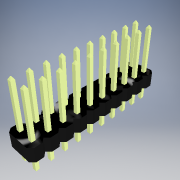
# Autodesk Inventor part: PinHeader-2x10-Male-NoCover
Saved by Autodesk Inventor 2018 (Build 220112000, 112)
## iProperties
Created: 2020-04-19
Part Number: PinHeader-2x10-Male-NoCover
Material: Všeobecné
Document SubType Name: Modeling
Designer: Jozko Mrkvicka
Density: 1 g/cm^3
Appearance: Výchozí
Author: Jozko Mrkvicka
Autodesk Inventor part; units mm, degrees
ref_plane "YZ Plane" through (0, 0, 0) normal (1, 0, 0) x (0, 1, 0)
ref_plane "XZ Plane" through (0, 0, 0) normal (0, 1, 0) x (-1, 0, 0)
ref_plane "XY Plane" through (0, 0, 0) normal (0, 0, 1) x (1, 0, 0)
sketch "Náčrt4" plane through (0, 0, 0) normal (0, 1, 0) x (-1, 0, 0)
  line L0 (4.445, 0) -> (0.635, 0)
  line L1 (0.635, -25.4) -> (4.445, -25.4)
  line L2 (4.445, 0) -> (5.08, -0.635)
  line L3 (5.08, -1.905) -> (4.445, -2.54)
  line L4 (4.445, -2.54) -> (5.08, -3.175)
  line L5 (5.08, -4.445) -> (4.445, -5.08)
  line L6 (4.445, -5.08) -> (5.08, -5.715)
  line L7 (5.08, -6.985) -> (4.445, -7.62)
  line L8 (4.445, -7.62) -> (5.08, -8.255)
  line L9 (5.08, -8.255) -> (5.08, -9.525)
  line L10 (5.08, -9.525) -> (4.445, -10.16)
  line L11 (4.445, -10.16) -> (5.08, -10.795)
  line L12 (5.08, -12.065) -> (4.445, -12.7)
  line L13 (4.445, -12.7) -> (5.08, -13.335)
  line L14 (5.08, -14.605) -> (4.445, -15.24)
  line L15 (4.445, -15.24) -> (5.08, -15.875)
  line L16 (5.08, -17.145) -> (4.445, -17.78)
  line L17 (4.445, -17.78) -> (5.08, -18.415)
  line L18 (5.08, -19.685) -> (4.445, -20.32)
  line L19 (4.445, -20.32) -> (5.08, -20.955)
  line L20 (5.08, -22.225) -> (4.445, -22.86)
  line L21 (4.445, -22.86) -> (5.08, -23.495)
  line L22 (5.08, -24.765) -> (4.445, -25.4)
  line L23 (5.08, -24.765) -> (5.08, -23.495)
  line L24 (5.08, -22.225) -> (5.08, -20.955)
  line L25 (5.08, -19.685) -> (5.08, -18.415)
  line L26 (5.08, -17.145) -> (5.08, -15.875)
  line L27 (5.08, -14.605) -> (5.08, -13.335)
  line L28 (5.08, -12.065) -> (5.08, -10.795)
  line L29 (5.08, -9.525) -> (5.08, -8.255)
  line L30 (5.08, -6.985) -> (5.08, -5.715)
  line L31 (5.08, -4.445) -> (5.08, -3.175)
  line L32 (5.08, -1.905) -> (5.08, -0.635)
  line L33 (0.635, 0) -> (0, -0.635)
  line L34 (0, -1.905) -> (0.635, -2.54)
  line L35 (0.635, -2.54) -> (0, -3.175)
  line L36 (0, -4.445) -> (0.635, -5.08)
  line L37 (0.635, -5.08) -> (0, -5.715)
  line L38 (0, -6.985) -> (0.635, -7.62)
  line L39 (0.635, -7.62) -> (0, -8.255)
  line L40 (0, -9.525) -> (0.635, -10.16)
  line L41 (0.635, -10.16) -> (0, -10.795)
  line L42 (0, -12.065) -> (0.635, -12.7)
  line L43 (0.635, -12.7) -> (0, -13.335)
  line L44 (0, -14.605) -> (0.635, -15.24)
  line L45 (0.635, -15.24) -> (0, -15.875)
  line L46 (0, -17.145) -> (0.635, -17.78)
  line L47 (0.635, -17.78) -> (0, -18.415)
  line L48 (0, -19.685) -> (0.635, -20.32)
  line L49 (0.635, -20.32) -> (0, -20.955)
  line L50 (0, -22.225) -> (0.635, -22.86)
  line L51 (0.635, -22.86) -> (0, -23.495)
  line L52 (0, -24.765) -> (0.635, -25.4)
  line L53 (0, -23.495) -> (0, -24.765)
  line L54 (0, -20.955) -> (0, -22.225)
  line L55 (0, -18.415) -> (0, -19.685)
  line L56 (0, -15.875) -> (0, -17.145)
  line L57 (0, -13.335) -> (0, -14.605)
  line L58 (0, -10.795) -> (0, -12.065)
  line L59 (0, -8.255) -> (0, -9.525)
  line L60 (0, -5.715) -> (0, -6.985)
  line L61 (0, -0.635) -> (0, -1.905)
  line L62 (0, -3.175) -> (0, -4.445)
  constraints: 126 end point, 102 parallel, 40 perpendicular, 1 horizontal
extrude "Vysunutí5" add sketch "Náčrt4" along normal blind 2.54
sketch "Náčrt5" plane through (0, 2.54, 0) normal (0, 1, 0) x (1, 0, 0)
  line L0 (-4.1275, 11.7475) -> (-4.1275, 11.1125)
  line L1 (-4.1275, 11.1125) -> (-3.4925, 11.1125)
  line L2 (-3.4925, 11.1125) -> (-3.4925, 11.7475)
  line L3 (-1.5875, 11.7475) -> (-1.5875, 11.1125)
  line L4 (-0.9525, 11.7475) -> (-1.5875, 11.7475)
  line L5 (-0.9525, 11.1125) -> (-0.9525, 11.7475)
  line L6 (-3.4925, 9.2075) -> (-4.1275, 9.2075)
  line L7 (-4.1275, 9.2075) -> (-4.1275, 8.5725)
  line L8 (-0.9525, 9.2075) -> (-1.5875, 9.2075)
  line L9 (-1.5875, 9.2075) -> (-1.5875, 8.5725)
  line L10 (-0.9525, 8.5725) -> (-0.9525, 9.2075)
  line L11 (-1.5875, 11.1125) -> (-0.9525, 11.1125)
  line L12 (-3.4925, 8.5725) -> (-3.4925, 9.2075)
  line L13 (-1.5875, 6.6675) -> (-1.5875, 6.0325)
  line L14 (-4.1275, 8.5725) -> (-3.4925, 8.5725)
  line L15 (-1.5875, 8.5725) -> (-0.9525, 8.5725)
  line L16 (-3.4925, 6.6675) -> (-4.1275, 6.6675)
  line L17 (-4.1275, 6.0325) -> (-3.4925, 6.0325)
  line L18 (-4.1275, 6.6675) -> (-4.1275, 6.0325)
  line L19 (-3.4925, 6.0325) -> (-3.4925, 6.6675)
  line L20 (-0.9525, 6.6675) -> (-1.5875, 6.6675)
  line L21 (-0.9525, 6.0325) -> (-0.9525, 6.6675)
  line L22 (-1.5875, 6.0325) -> (-0.9525, 6.0325)
  line L23 (-0.9525, 4.1275) -> (-1.5875, 4.1275)
  line L24 (-1.5875, 4.1275) -> (-1.5875, 3.4925)
  line L25 (-1.5875, 3.4925) -> (-0.9525, 3.4925)
  line L26 (-0.9525, 3.4925) -> (-0.9525, 4.1275)
  line L27 (-4.1275, 4.1275) -> (-4.1275, 3.4925)
  line L28 (-4.1275, 3.4925) -> (-3.4925, 3.4925)
  line L29 (-3.4925, 3.4925) -> (-3.4925, 4.1275)
  line L30 (-3.4925, 4.1275) -> (-4.1275, 4.1275)
  line L31 (-0.9525, 1.5875) -> (-1.5875, 1.5875)
  line L32 (-3.4925, 1.5875) -> (-4.1275, 1.5875)
  line L33 (-1.5875, 1.5875) -> (-1.5875, 0.9525)
  line L34 (-1.5875, 0.9525) -> (-0.9525, 0.9525)
  line L35 (-0.9525, 0.9525) -> (-0.9525, 1.5875)
  line L36 (-4.1275, 1.5875) -> (-4.1275, 0.9525)
  line L37 (-4.1275, 0.9525) -> (-3.4925, 0.9525)
  line L38 (-3.4925, 0.9525) -> (-3.4925, 1.5875)
  line L39 (-3.4925, 11.7475) -> (-4.1275, 11.7475)
  line L40 (-0.9525, 14.2875) -> (-1.5875, 14.2875)
  line L41 (-0.9525, 13.6525) -> (-0.9525, 14.2875)
  line L42 (-1.5875, 13.6525) -> (-0.9525, 13.6525)
  line L43 (-1.5875, 14.2875) -> (-1.5875, 13.6525)
  line L44 (-3.4925, 14.2875) -> (-4.1275, 14.2875)
  line L45 (-3.4925, 13.6525) -> (-3.4925, 14.2875)
  line L46 (-4.1275, 14.2875) -> (-4.1275, 13.6525)
  line L47 (-4.1275, 13.6525) -> (-3.4925, 13.6525)
  line L48 (-4.1275, 24.4475) -> (-4.1275, 23.8125)
  line L49 (-4.1275, 23.8125) -> (-3.4925, 23.8125)
  line L50 (-3.4925, 23.8125) -> (-3.4925, 24.4475)
  line L51 (-1.5875, 24.4475) -> (-1.5875, 23.8125)
  line L52 (-0.9525, 24.4475) -> (-1.5875, 24.4475)
  line L53 (-0.9525, 23.8125) -> (-0.9525, 24.4475)
  line L54 (-1.5875, 21.2725) -> (-0.9525, 21.2725)
  line L55 (-4.1275, 21.2725) -> (-3.4925, 21.2725)
  line L56 (-0.9525, 21.9075) -> (-1.5875, 21.9075)
  line L57 (-1.5875, 21.9075) -> (-1.5875, 21.2725)
  line L58 (-0.9525, 21.2725) -> (-0.9525, 21.9075)
  line L59 (-1.5875, 23.8125) -> (-0.9525, 23.8125)
  line L60 (-3.4925, 21.9075) -> (-4.1275, 21.9075)
  line L61 (-4.1275, 21.9075) -> (-4.1275, 21.2725)
  line L62 (-3.4925, 24.4475) -> (-4.1275, 24.4475)
  line L63 (-3.4925, 21.2725) -> (-3.4925, 21.9075)
  line L64 (-4.1275, 16.1925) -> (-3.4925, 16.1925)
  line L65 (-3.4925, 16.8275) -> (-4.1275, 16.8275)
  line L66 (-4.1275, 16.8275) -> (-4.1275, 16.1925)
  line L67 (-3.4925, 16.1925) -> (-3.4925, 16.8275)
  line L68 (-1.5875, 16.8275) -> (-1.5875, 16.1925)
  line L69 (-1.5875, 16.1925) -> (-0.9525, 16.1925)
  line L70 (-0.9525, 16.8275) -> (-1.5875, 16.8275)
  line L71 (-0.9525, 16.1925) -> (-0.9525, 16.8275)
  line L72 (-3.4925, 19.3675) -> (-4.1275, 19.3675)
  line L73 (-4.1275, 18.7325) -> (-3.4925, 18.7325)
  line L74 (-4.1275, 19.3675) -> (-4.1275, 18.7325)
  line L75 (-3.4925, 18.7325) -> (-3.4925, 19.3675)
  line L76 (-0.9525, 19.3675) -> (-1.5875, 19.3675)
  line L77 (-1.5875, 19.3675) -> (-1.5875, 18.7325)
  line L78 (-0.9525, 18.7325) -> (-0.9525, 19.3675)
  line L79 (-1.5875, 18.7325) -> (-0.9525, 18.7325)
  point P0 (0, 0)
  point P1 (-3.81, 1.27)
  point P2 (-3.81, 13.97)
  constraints: 160 end point
extrude "Vysunutí6" add sketch "Náčrt5" along normal blind 8.255
sketch "Náčrt6" plane through (0, 0, 0) normal (0, -1, 0) x (1, 0, 0)
  line L0 (-4.1275, -19.3675) -> (-3.4925, -19.3675) projected
  line L1 (-3.4925, -19.3675) -> (-3.4925, -18.7325) projected
  line L2 (-3.4925, -18.7325) -> (-4.1275, -18.7325) projected
  line L3 (-4.1275, -18.7325) -> (-4.1275, -19.3675) projected
  line L4 (-1.5875, -16.8275) -> (-0.9525, -16.8275) projected
  line L5 (-0.9525, -16.8275) -> (-0.9525, -16.1925) projected
  line L6 (-0.9525, -16.1925) -> (-1.5875, -16.1925) projected
  line L7 (-1.5875, -16.1925) -> (-1.5875, -16.8275) projected
  line L8 (-1.5875, -21.9075) -> (-0.9525, -21.9075) projected
  line L9 (-0.9525, -21.9075) -> (-0.9525, -21.2725) projected
  line L10 (-0.9525, -21.2725) -> (-1.5875, -21.2725) projected
  line L11 (-1.5875, -21.2725) -> (-1.5875, -21.9075) projected
  line L12 (-4.1275, -24.4475) -> (-3.4925, -24.4475) projected
  line L13 (-3.4925, -24.4475) -> (-3.4925, -23.8125) projected
  line L14 (-3.4925, -23.8125) -> (-4.1275, -23.8125) projected
  line L15 (-4.1275, -23.8125) -> (-4.1275, -24.4475) projected
  line L16 (-1.5875, -14.2875) -> (-0.9525, -14.2875) projected
  line L17 (-0.9525, -14.2875) -> (-0.9525, -13.6525) projected
  line L18 (-0.9525, -13.6525) -> (-1.5875, -13.6525) projected
  line L19 (-1.5875, -13.6525) -> (-1.5875, -14.2875) projected
  line L20 (-4.1275, -6.6675) -> (-3.4925, -6.6675) projected
  line L21 (-3.4925, -6.6675) -> (-3.4925, -6.0325) projected
  line L22 (-3.4925, -6.0325) -> (-4.1275, -6.0325) projected
  line L23 (-4.1275, -6.0325) -> (-4.1275, -6.6675) projected
  line L24 (-4.1275, -4.1275) -> (-3.4925, -4.1275) projected
  line L25 (-3.4925, -4.1275) -> (-3.4925, -3.4925) projected
  line L26 (-3.4925, -3.4925) -> (-4.1275, -3.4925) projected
  line L27 (-4.1275, -3.4925) -> (-4.1275, -4.1275) projected
  line L28 (-4.1275, -9.2075) -> (-3.4925, -9.2075) projected
  line L29 (-3.4925, -9.2075) -> (-3.4925, -8.5725) projected
  line L30 (-3.4925, -8.5725) -> (-4.1275, -8.5725) projected
  line L31 (-4.1275, -8.5725) -> (-4.1275, -9.2075) projected
  line L32 (-1.5875, -11.7475) -> (-0.9525, -11.7475) projected
  line L33 (-0.9525, -11.7475) -> (-0.9525, -11.1125) projected
  line L34 (-0.9525, -11.1125) -> (-1.5875, -11.1125) projected
  line L35 (-1.5875, -11.1125) -> (-1.5875, -11.7475) projected
  line L36 (-1.5875, -1.5875) -> (-0.9525, -1.5875) projected
  line L37 (-0.9525, -1.5875) -> (-0.9525, -0.9525) projected
  line L38 (-0.9525, -0.9525) -> (-1.5875, -0.9525) projected
  line L39 (-1.5875, -0.9525) -> (-1.5875, -1.5875) projected
  line L40 (-3.4925, -0.9525) -> (-4.1275, -0.9525) projected
  line L41 (-4.1275, -0.9525) -> (-4.1275, -1.5875) projected
  line L42 (-4.1275, -1.5875) -> (-3.4925, -1.5875) projected
  line L43 (-3.4925, -1.5875) -> (-3.4925, -0.9525) projected
  line L44 (-4.1275, -11.7475) -> (-3.4925, -11.7475) projected
  line L45 (-3.4925, -11.7475) -> (-3.4925, -11.1125) projected
  line L46 (-3.4925, -11.1125) -> (-4.1275, -11.1125) projected
  line L47 (-4.1275, -11.1125) -> (-4.1275, -11.7475) projected
  line L48 (-1.5875, -9.2075) -> (-0.9525, -9.2075) projected
  line L49 (-0.9525, -9.2075) -> (-0.9525, -8.5725) projected
  line L50 (-0.9525, -8.5725) -> (-1.5875, -8.5725) projected
  line L51 (-1.5875, -8.5725) -> (-1.5875, -9.2075) projected
  line L52 (-1.5875, -4.1275) -> (-0.9525, -4.1275) projected
  line L53 (-0.9525, -4.1275) -> (-0.9525, -3.4925) projected
  line L54 (-0.9525, -3.4925) -> (-1.5875, -3.4925) projected
  line L55 (-1.5875, -3.4925) -> (-1.5875, -4.1275) projected
  line L56 (-1.5875, -6.6675) -> (-0.9525, -6.6675) projected
  line L57 (-0.9525, -6.6675) -> (-0.9525, -6.0325) projected
  line L58 (-0.9525, -6.0325) -> (-1.5875, -6.0325) projected
  line L59 (-1.5875, -6.0325) -> (-1.5875, -6.6675) projected
  line L60 (-1.5875, -24.4475) -> (-0.9525, -24.4475) projected
  line L61 (-0.9525, -24.4475) -> (-0.9525, -23.8125) projected
  line L62 (-0.9525, -23.8125) -> (-1.5875, -23.8125) projected
  line L63 (-1.5875, -23.8125) -> (-1.5875, -24.4475) projected
  line L64 (-4.1275, -21.9075) -> (-3.4925, -21.9075) projected
  line L65 (-3.4925, -21.9075) -> (-3.4925, -21.2725) projected
  line L66 (-3.4925, -21.2725) -> (-4.1275, -21.2725) projected
  line L67 (-4.1275, -21.2725) -> (-4.1275, -21.9075) projected
  line L68 (-4.1275, -13.6525) -> (-4.1275, -14.2875) projected
  line L69 (-4.1275, -14.2875) -> (-3.4925, -14.2875) projected
  line L70 (-3.4925, -14.2875) -> (-3.4925, -13.6525) projected
  line L71 (-3.4925, -13.6525) -> (-4.1275, -13.6525) projected
  line L72 (-4.1275, -16.1925) -> (-4.1275, -16.8275) projected
  line L73 (-4.1275, -16.8275) -> (-3.4925, -16.8275) projected
  line L74 (-3.4925, -16.8275) -> (-3.4925, -16.1925) projected
  line L75 (-3.4925, -16.1925) -> (-4.1275, -16.1925) projected
  line L76 (-0.9525, -18.7325) -> (-1.5875, -18.7325) projected
  line L77 (-1.5875, -18.7325) -> (-1.5875, -19.3675) projected
  line L78 (-1.5875, -19.3675) -> (-0.9525, -19.3675) projected
  line L79 (-0.9525, -19.3675) -> (-0.9525, -18.7325) projected
  line L80 (-4.445, 0) -> (-0.635, 0) projected
  line L81 (-0.635, 0) -> (0, -0.635) projected
  line L82 (0, -0.635) -> (0, -1.905) projected
  line L83 (0, -1.905) -> (-0.635, -2.54) projected
  line L84 (-0.635, -2.54) -> (0, -3.175) projected
  line L85 (0, -3.175) -> (0, -4.445) projected
  line L86 (0, -4.445) -> (-0.635, -5.08) projected
  line L87 (-0.635, -5.08) -> (0, -5.715) projected
  line L88 (0, -5.715) -> (0, -6.985) projected
  line L89 (0, -6.985) -> (-0.635, -7.62) projected
  line L90 (-0.635, -7.62) -> (0, -8.255) projected
  line L91 (0, -8.255) -> (0, -9.525) projected
  line L92 (0, -9.525) -> (-0.635, -10.16) projected
  line L93 (-0.635, -10.16) -> (0, -10.795) projected
  line L94 (0, -10.795) -> (0, -12.065) projected
  line L95 (0, -12.065) -> (-0.635, -12.7) projected
  line L96 (-0.635, -12.7) -> (0, -13.335) projected
  line L97 (0, -13.335) -> (0, -14.605) projected
  line L98 (0, -14.605) -> (-0.635, -15.24) projected
  line L99 (-0.635, -15.24) -> (0, -15.875) projected
  line L100 (0, -15.875) -> (0, -17.145) projected
  line L101 (0, -17.145) -> (-0.635, -17.78) projected
  line L102 (-0.635, -17.78) -> (0, -18.415) projected
  line L103 (0, -18.415) -> (0, -19.685) projected
  line L104 (0, -19.685) -> (-0.635, -20.32) projected
  line L105 (-0.635, -20.32) -> (0, -20.955) projected
  line L106 (0, -20.955) -> (0, -22.225) projected
  line L107 (0, -22.225) -> (-0.635, -22.86) projected
  line L108 (-0.635, -22.86) -> (0, -23.495) projected
  line L109 (0, -23.495) -> (0, -24.765) projected
  line L110 (0, -24.765) -> (-0.635, -25.4) projected
  line L111 (-0.635, -25.4) -> (-4.445, -25.4) projected
  line L112 (-4.445, -25.4) -> (-5.08, -24.765) projected
  line L113 (-5.08, -24.765) -> (-5.08, -23.495) projected
  line L114 (-5.08, -23.495) -> (-4.445, -22.86) projected
  line L115 (-4.445, -22.86) -> (-5.08, -22.225) projected
  line L116 (-5.08, -22.225) -> (-5.08, -20.955) projected
  line L117 (-5.08, -20.955) -> (-4.445, -20.32) projected
  line L118 (-4.445, -20.32) -> (-5.08, -19.685) projected
  line L119 (-5.08, -19.685) -> (-5.08, -18.415) projected
  line L120 (-5.08, -18.415) -> (-4.445, -17.78) projected
  line L121 (-4.445, -17.78) -> (-5.08, -17.145) projected
  line L122 (-5.08, -17.145) -> (-5.08, -15.875) projected
  line L123 (-5.08, -15.875) -> (-4.445, -15.24) projected
  line L124 (-4.445, -15.24) -> (-5.08, -14.605) projected
  line L125 (-5.08, -14.605) -> (-5.08, -13.335) projected
  line L126 (-5.08, -13.335) -> (-4.445, -12.7) projected
  line L127 (-4.445, -12.7) -> (-5.08, -12.065) projected
  line L128 (-5.08, -12.065) -> (-5.08, -10.795) projected
  line L129 (-5.08, -10.795) -> (-4.445, -10.16) projected
  line L130 (-4.445, -10.16) -> (-5.08, -9.525) projected
  line L131 (-5.08, -9.525) -> (-5.08, -8.255) projected
  line L132 (-5.08, -8.255) -> (-4.445, -7.62) projected
  line L133 (-4.445, -7.62) -> (-5.08, -6.985) projected
  line L134 (-5.08, -6.985) -> (-5.08, -5.715) projected
  line L135 (-5.08, -5.715) -> (-4.445, -5.08) projected
  line L136 (-4.445, -5.08) -> (-5.08, -4.445) projected
  line L137 (-5.08, -4.445) -> (-5.08, -3.175) projected
  line L138 (-5.08, -3.175) -> (-4.445, -2.54) projected
  line L139 (-4.445, -2.54) -> (-5.08, -1.905) projected
  line L140 (-5.08, -1.905) -> (-5.08, -0.635) projected
  line L141 (-5.08, -0.635) -> (-4.445, 0) projected
  point P0 (0, 0)
extrude "Vysunutí7" add sketch "Náčrt6" along normal blind 3.175 contours L3 L2 L1 L0 | L7 L6 L5 L4 | L11 L10 L9 L8 | L15 L14 L13 L12 | L19 L18 L17 L16 | L23 L22 L21 L20 | L27 L26 L25 L24 | L31 L30 L29 L28 | L35 L34 L33 L32 | L39 L38 L37 L36 | L43 L42 L41 L40 | L47 L46 L45 L44 | L51 L50 L49 L48 | L55 L54 L53 L52 | L59 L58 L57 L56 | L63 L62 L61 L60 | L67 L66 L65 L64 | L71 L70 L69 L68 | L75 L74 L73 L72 | L79 L78 L77 L76
chamfer "Zkosení21" distance 0.254 angle 60 4 edges at (-4.1275, -3.175, -24.13) (-3.81, -3.175, -23.8125) (-3.4925, -3.175, -24.13) (-3.81, -3.175, -24.4475) measured on face at (-3.9158, -3.175, -24.0242)
chamfer "Zkosení22" distance 0.254 angle 60 4 edges at (-1.27, -3.175, -23.8125) (-1.5875, -3.175, -24.13) (-0.9525, -3.175, -24.13) (-1.27, -3.175, -24.4475) measured on face at (-1.3758, -3.175, -24.0242)
chamfer "Zkosení23" distance 0.254 angle 60 4 edges at (-1.5875, -3.175, -21.59) (-1.27, -3.175, -21.9075) (-0.9525, -3.175, -21.59) (-1.27, -3.175, -21.2725) measured on face at (-1.3758, -3.175, -21.4842)
chamfer "Zkosení24" distance 0.254 angle 60 4 edges at (-3.81, -3.175, -21.2725) (-4.1275, -3.175, -21.59) (-3.4925, -3.175, -21.59) (-3.81, -3.175, -21.9075) measured on face at (-3.9158, -3.175, -21.4842)
chamfer "Zkosení25" distance 0.254 angle 60 4 edges at (-1.5875, -3.175, -19.05) (-1.27, -3.175, -18.7325) (-0.9525, -3.175, -19.05) (-1.27, -3.175, -19.3675) measured on face at (-1.3758, -3.175, -18.9442)
chamfer "Zkosení26" distance 0.254 angle 60 4 edges at (-4.1275, -3.175, -19.05) (-3.81, -3.175, -18.7325) (-3.4925, -3.175, -19.05) (-3.81, -3.175, -19.3675) measured on face at (-3.9158, -3.175, -18.9442)
chamfer "Zkosení27" distance 0.254 angle 60 4 edges at (-4.1275, -3.175, -16.51) (-3.81, -3.175, -16.1925) (-3.4925, -3.175, -16.51) (-3.81, -3.175, -16.8275) measured on face at (-3.9158, -3.175, -16.4042)
chamfer "Zkosení28" distance 0.254 angle 60 4 edges at (-1.5875, -3.175, -16.51) (-1.27, -3.175, -16.1925) (-0.9525, -3.175, -16.51) (-1.27, -3.175, -16.8275) measured on face at (-1.3758, -3.175, -16.4042)
chamfer "Zkosení29" distance 0.254 angle 60 4 edges at (-4.1275, -3.175, -13.97) (-3.81, -3.175, -13.6525) (-3.4925, -3.175, -13.97) (-3.81, -3.175, -14.2875) measured on face at (-3.9158, -3.175, -13.8642)
chamfer "Zkosení30" distance 0.254 angle 60 4 edges at (-1.5875, -3.175, -13.97) (-0.9525, -3.175, -13.97) (-1.27, -3.175, -13.6525) (-1.27, -3.175, -14.2875) measured on face at (-1.3758, -3.175, -13.8642)
chamfer "Zkosení31" distance 0.254 angle 60 4 edges at (-4.1275, -3.175, -11.43) (-3.81, -3.175, -11.1125) (-3.4925, -3.175, -11.43) (-3.81, -3.175, -11.7475) measured on face at (-3.9158, -3.175, -11.3242)
chamfer "Zkosení32" distance 0.254 angle 60 4 edges at (-1.5875, -3.175, -11.43) (-1.27, -3.175, -11.1125) (-0.9525, -3.175, -11.43) (-1.27, -3.175, -11.7475) measured on face at (-1.3758, -3.175, -11.3242)
chamfer "Zkosení33" distance 0.254 angle 60 4 edges at (-1.5875, -3.175, -8.89) (-1.27, -3.175, -8.5725) (-0.9525, -3.175, -8.89) (-1.27, -3.175, -9.2075) measured on face at (-1.3758, -3.175, -8.7842)
chamfer "Zkosení34" distance 0.254 angle 60 4 edges at (-4.1275, -3.175, -8.89) (-3.81, -3.175, -8.5725) (-3.4925, -3.175, -8.89) (-3.81, -3.175, -9.2075) measured on face at (-3.9158, -3.175, -8.7842)
chamfer "Zkosení35" distance 0.254 angle 60 4 edges at (-1.27, -3.175, -6.0325) (-1.5875, -3.175, -6.35) (-1.27, -3.175, -6.6675) (-0.9525, -3.175, -6.35) measured on face at (-1.3758, -3.175, -6.2442)
chamfer "Zkosení36" distance 0.254 angle 60 4 edges at (-4.1275, -3.175, -6.35) (-3.81, -3.175, -6.0325) (-3.4925, -3.175, -6.35) (-3.81, -3.175, -6.6675) measured on face at (-3.9158, -3.175, -6.2442)
chamfer "Zkosení37" distance 0.254 angle 60 4 edges at (-4.1275, -3.175, -3.81) (-3.81, -3.175, -3.4925) (-3.4925, -3.175, -3.81) (-3.81, -3.175, -4.1275) measured on face at (-3.9158, -3.175, -3.7042)
chamfer "Zkosení38" distance 0.254 angle 60 4 edges at (-1.5875, -3.175, -3.81) (-1.27, -3.175, -3.4925) (-0.9525, -3.175, -3.81) (-1.27, -3.175, -4.1275) measured on face at (-1.3758, -3.175, -3.7042)
chamfer "Zkosení39" distance 0.254 angle 60 4 edges at (-1.27, -3.175, -0.9525) (-0.9525, -3.175, -1.27) (-1.27, -3.175, -1.5875) (-1.5875, -3.175, -1.27) measured on face at (-1.3758, -3.175, -1.1642)
chamfer "Zkosení40" distance 0.254 angle 60 4 edges at (-3.4925, -3.175, -1.27) (-3.81, -3.175, -0.9525) (-3.81, -3.175, -1.5875) (-4.1275, -3.175, -1.27) measured on face at (-3.9158, -3.175, -1.1642)
chamfer "Zkosení41" distance 0.254 angle 60 4 edges at (-1.27, 10.795, -1.5875) (-1.5875, 10.795, -1.27) (-0.9525, 10.795, -1.27) (-1.27, 10.795, -0.9525) measured on face at (-1.3758, 10.795, -1.3758)
chamfer "Zkosení42" distance 0.254 angle 60 4 edges at (-4.1275, 10.795, -1.27) (-3.4925, 10.795, -1.27) (-3.81, 10.795, -1.5875) (-3.81, 10.795, -0.9525) measured on face at (-3.9158, 10.795, -1.3758)
chamfer "Zkosení43" distance 0.254 angle 60 4 edges at (-1.27, 10.795, -4.1275) (-1.5875, 10.795, -3.81) (-1.27, 10.795, -3.4925) (-0.9525, 10.795, -3.81) measured on face at (-1.3758, 10.795, -3.9158)
chamfer "Zkosení44" distance 0.254 angle 60 4 edges at (-3.4925, 10.795, -3.81) (-3.81, 10.795, -4.1275) (-4.1275, 10.795, -3.81) (-3.81, 10.795, -3.4925) measured on face at (-3.9158, 10.795, -3.9158)
chamfer "Zkosení45" distance 0.254 angle 60 4 edges at (-1.27, 10.795, -6.6675) (-1.5875, 10.795, -6.35) (-1.27, 10.795, -6.0325) (-0.9525, 10.795, -6.35) measured on face at (-1.3758, 10.795, -6.4558)
chamfer "Zkosení46" distance 0.254 angle 60 4 edges at (-4.1275, 10.795, -6.35) (-3.4925, 10.795, -6.35) (-3.81, 10.795, -6.6675) (-3.81, 10.795, -6.0325) measured on face at (-3.9158, 10.795, -6.4558)
chamfer "Zkosení47" distance 0.254 angle 60 4 edges at (-1.27, 10.795, -9.2075) (-1.5875, 10.795, -8.89) (-1.27, 10.795, -8.5725) (-0.9525, 10.795, -8.89) measured on face at (-1.3758, 10.795, -8.9958)
chamfer "Zkosení48" distance 0.254 angle 60 4 edges at (-4.1275, 10.795, -8.89) (-3.4925, 10.795, -8.89) (-3.81, 10.795, -9.2075) (-3.81, 10.795, -8.5725) measured on face at (-3.9158, 10.795, -8.9958)
chamfer "Zkosení49" distance 0.254 angle 60 4 edges at (-1.5875, 10.795, -11.43) (-1.27, 10.795, -11.7475) (-0.9525, 10.795, -11.43) (-1.27, 10.795, -11.1125) measured on face at (-1.3758, 10.795, -11.5358)
chamfer "Zkosení50" distance 0.254 angle 60 4 edges at (-4.1275, 10.795, -11.43) (-3.4925, 10.795, -11.43) (-3.81, 10.795, -11.7475) (-3.81, 10.795, -11.1125) measured on face at (-3.9158, 10.795, -11.5358)
chamfer "Zkosení51" distance 0.254 angle 60 4 edges at (-1.27, 10.795, -14.2875) (-0.9525, 10.795, -13.97) (-1.27, 10.795, -13.6525) (-1.5875, 10.795, -13.97) measured on face at (-1.3758, 10.795, -14.0758)
chamfer "Zkosení52" distance 0.254 angle 60 4 edges at (-4.1275, 10.795, -13.97) (-3.4925, 10.795, -13.97) (-3.81, 10.795, -14.2875) (-3.81, 10.795, -13.6525) measured on face at (-3.7042, 10.795, -13.8642)
chamfer "Zkosení53" distance 0.254 angle 60 4 edges at (-1.27, 10.795, -16.8275) (-1.27, 10.795, -16.1925) (-0.9525, 10.795, -16.51) (-1.5875, 10.795, -16.51) measured on face at (-1.3758, 10.795, -16.6158)
chamfer "Zkosení54" distance 0.254 angle 60 4 edges at (-4.1275, 10.795, -16.51) (-3.81, 10.795, -16.8275) (-3.4925, 10.795, -16.51) (-3.81, 10.795, -16.1925) measured on face at (-3.7042, 10.795, -16.4042)
chamfer "Zkosení55" distance 0.254 angle 60 4 edges at (-1.27, 10.795, -19.3675) (-1.5875, 10.795, -19.05) (-1.27, 10.795, -18.7325) (-0.9525, 10.795, -19.05) measured on face at (-1.3758, 10.795, -19.1558)
chamfer "Zkosení56" distance 0.254 angle 60 4 edges at (-3.81, 10.795, -19.3675) (-4.1275, 10.795, -19.05) (-3.81, 10.795, -18.7325) (-3.4925, 10.795, -19.05) measured on face at (-3.9158, 10.795, -19.1558)
chamfer "Zkosení57" distance 0.254 angle 60 4 edges at (-1.5875, 10.795, -21.59) (-0.9525, 10.795, -21.59) (-1.27, 10.795, -21.9075) (-1.27, 10.795, -21.2725) measured on face at (-1.3758, 10.795, -21.6958)
chamfer "Zkosení58" distance 0.254 angle 60 4 edges at (-3.81, 10.795, -21.9075) (-3.81, 10.795, -21.2725) (-4.1275, 10.795, -21.59) (-3.4925, 10.795, -21.59) measured on face at (-3.9158, 10.795, -21.6958)
chamfer "Zkosení59" distance 0.254 angle 60 4 edges at (-1.5875, 10.795, -24.13) (-1.27, 10.795, -23.8125) (-1.27, 10.795, -24.4475) (-0.9525, 10.795, -24.13) measured on face at (-1.3758, 10.795, -24.2358)
chamfer "Zkosení60" distance 0.254 angle 60 4 edges at (-4.1275, 10.795, -24.13) (-3.81, 10.795, -23.8125) (-3.81, 10.795, -24.4475) (-3.4925, 10.795, -24.13) measured on face at (-3.9158, 10.795, -24.2358)
